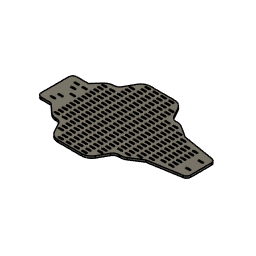
Old_Electronics plate v1 (Autodesk Fusion 360 design; units mm, degrees)
Autodesk Fusion 360 part; units mm, degrees
note: some values were not read from the file. Set by a fixed rule: which sketch regions a step uses.
(part 1 of 4)
sketch "Sketch2" plane through (0, 0, 0) normal (0, 1, 0) x (1, 0, 0)
  line L0 (270, -122.5) -> (360, -107.5)
  line L1 (360, -37.5) -> (270, -22.5)
  line L2 (360, -37.5) -> (360, -107.5)
  line L3 (270, -122.5) -> (235, -145)
  line L4 (235, 0) -> (270, -22.5)
  line L5 (-10, -27.5) -> (-10, -117.5)
  line L6 (55, -145) -> (25, -117.5)
  line L7 (25, -117.5) -> (-10, -117.5)
  line L8 (-10, -27.5) -> (29.7917, -27.5)
  line L9 (348.5, -55) -> (338.5, -55)
  line L10 (338.5, -58) -> (348.5, -58)
  arc A0 (338.5, -55) -> (338.5, -58) centre (338.5, -56.5) ccw
  arc A1 (348.5, -58) -> (348.5, -55) centre (348.5, -56.5) ccw
  line L11 (338.5, -87) -> (348.5, -87)
  arc A2 (338.5, -87) -> (338.5, -90) centre (338.5, -88.5) ccw
  line L12 (348.5, -90) -> (338.5, -90)
  arc A3 (348.5, -90) -> (348.5, -87) centre (348.5, -88.5) ccw
  line L13 (25, -55) -> (15, -55)
  arc A4 (15, -55) -> (15, -58) centre (15, -56.5) ccw
  line L14 (15, -58) -> (25, -58)
  arc A5 (25, -58) -> (25, -55) centre (25, -56.5) ccw
  line L15 (25, -90) -> (15, -90)
  line L16 (15, -87) -> (25, -87)
  arc A6 (25, -90) -> (25, -87) centre (25, -88.5) ccw
  arc A7 (15, -87) -> (15, -90) centre (15, -88.5) ccw
  line L17 (180, -71) -> (170, -71)
  line L18 (170, -74) -> (180, -74)
  arc A8 (170, -71) -> (170, -74) centre (170, -72.5) ccw
  arc A9 (180, -74) -> (180, -71) centre (180, -72.5) ccw
  arc A10 (120, -184) -> (120, -181) centre (120, -182.5) ccw
  line L19 (120, -181) -> (110, -181)
  line L20 (110, -184) -> (120, -184)
  arc A11 (110, -181) -> (110, -184) centre (110, -182.5) ccw
  arc A12 (140, -184) -> (140, -181) centre (140, -182.5) ccw
  line L21 (140, -181) -> (130, -181)
  line L22 (130, -184) -> (140, -184)
  arc A13 (130, -181) -> (130, -184) centre (130, -182.5) ccw
  arc A14 (160, -184) -> (160, -181) centre (160, -182.5) ccw
  line L23 (160, -181) -> (150, -181)
  line L24 (150, -184) -> (160, -184)
  arc A15 (150, -181) -> (150, -184) centre (150, -182.5) ccw
  arc A16 (180, -184) -> (180, -181) centre (180, -182.5) ccw
  line L25 (180, -181) -> (170, -181)
  line L26 (170, -184) -> (180, -184)
  arc A17 (170, -181) -> (170, -184) centre (170, -182.5) ccw
  arc A18 (120, -174) -> (120, -171) centre (120, -172.5) ccw
  line L27 (120, -171) -> (110, -171)
  line L28 (110, -174) -> (120, -174)
  arc A19 (110, -171) -> (110, -174) centre (110, -172.5) ccw
  arc A20 (140, -174) -> (140, -171) centre (140, -172.5) ccw
  line L29 (140, -171) -> (130, -171)
  line L30 (130, -174) -> (140, -174)
  arc A21 (130, -171) -> (130, -174) centre (130, -172.5) ccw
  arc A22 (160, -174) -> (160, -171) centre (160, -172.5) ccw
  line L31 (160, -171) -> (150, -171)
  line L32 (150, -174) -> (160, -174)
  arc A23 (150, -171) -> (150, -174) centre (150, -172.5) ccw
  arc A24 (180, -174) -> (180, -171) centre (180, -172.5) ccw
  line L33 (180, -171) -> (170, -171)
  line L34 (170, -174) -> (180, -174)
  arc A25 (170, -171) -> (170, -174) centre (170, -172.5) ccw
  arc A26 (100, -164) -> (100, -161) centre (100, -162.5) ccw
  line L35 (100, -161) -> (90, -161)
  line L36 (90, -164) -> (100, -164)
  arc A27 (90, -161) -> (90, -164) centre (90, -162.5) ccw
  arc A28 (120, -164) -> (120, -161) centre (120, -162.5) ccw
  line L37 (120, -161) -> (110, -161)
  line L38 (110, -164) -> (120, -164)
  arc A29 (110, -161) -> (110, -164) centre (110, -162.5) ccw
  arc A30 (140, -164) -> (140, -161) centre (140, -162.5) ccw
  line L39 (140, -161) -> (130, -161)
  line L40 (130, -164) -> (140, -164)
  arc A31 (130, -161) -> (130, -164) centre (130, -162.5) ccw
  arc A32 (160, -164) -> (160, -161) centre (160, -162.5) ccw
  line L41 (160, -161) -> (150, -161)
  line L42 (150, -164) -> (160, -164)
  arc A33 (150, -161) -> (150, -164) centre (150, -162.5) ccw
  arc A34 (180, -164) -> (180, -161) centre (180, -162.5) ccw
  line L43 (180, -161) -> (170, -161)
  line L44 (170, -164) -> (180, -164)
  arc A35 (170, -161) -> (170, -164) centre (170, -162.5) ccw
  arc A36 (200, -164) -> (200, -161) centre (200, -162.5) ccw
  line L45 (200, -161) -> (190, -161)
  line L46 (190, -164) -> (200, -164)
  arc A37 (190, -161) -> (190, -164) centre (190, -162.5) ccw
  arc A38 (100, -154) -> (100, -151) centre (100, -152.5) ccw
  line L47 (100, -151) -> (90, -151)
  line L48 (90, -154) -> (100, -154)
  arc A39 (90, -151) -> (90, -154) centre (90, -152.5) ccw
  arc A40 (120, -154) -> (120, -151) centre (120, -152.5) ccw
  line L49 (120, -151) -> (110, -151)
  line L50 (110, -154) -> (120, -154)
  arc A41 (110, -151) -> (110, -154) centre (110, -152.5) ccw
  arc A42 (140, -154) -> (140, -151) centre (140, -152.5) ccw
  line L51 (140, -151) -> (130, -151)
  line L52 (130, -154) -> (140, -154)
  arc A43 (130, -151) -> (130, -154) centre (130, -152.5) ccw
  arc A44 (160, -154) -> (160, -151) centre (160, -152.5) ccw
  line L53 (160, -151) -> (150, -151)
  line L54 (150, -154) -> (160, -154)
  arc A45 (150, -151) -> (150, -154) centre (150, -152.5) ccw
  arc A46 (180, -154) -> (180, -151) centre (180, -152.5) ccw
  line L55 (180, -151) -> (170, -151)
  line L56 (170, -154) -> (180, -154)
  arc A47 (170, -151) -> (170, -154) centre (170, -152.5) ccw
  arc A48 (200, -154) -> (200, -151) centre (200, -152.5) ccw
  line L57 (200, -151) -> (190, -151)
  line L58 (190, -154) -> (200, -154)
  arc A49 (190, -151) -> (190, -154) centre (190, -152.5) ccw
  arc A50 (100, -144) -> (100, -141) centre (100, -142.5) ccw
  line L59 (100, -141) -> (90, -141)
  line L60 (90, -144) -> (100, -144)
  arc A51 (90, -141) -> (90, -144) centre (90, -142.5) ccw
  arc A52 (120, -144) -> (120, -141) centre (120, -142.5) ccw
  line L61 (120, -141) -> (110, -141)
  line L62 (110, -144) -> (120, -144)
  arc A53 (110, -141) -> (110, -144) centre (110, -142.5) ccw
  arc A54 (140, -144) -> (140, -141) centre (140, -142.5) ccw
  line L63 (140, -141) -> (130, -141)
  line L64 (130, -144) -> (140, -144)
  arc A55 (130, -141) -> (130, -144) centre (130, -142.5) ccw
  arc A56 (160, -144) -> (160, -141) centre (160, -142.5) ccw
  line L65 (160, -141) -> (150, -141)
  line L66 (150, -144) -> (160, -144)
  arc A57 (150, -141) -> (150, -144) centre (150, -142.5) ccw
  arc A58 (180, -144) -> (180, -141) centre (180, -142.5) ccw
  line L67 (180, -141) -> (170, -141)
  line L68 (170, -144) -> (180, -144)
  arc A59 (170, -141) -> (170, -144) centre (170, -142.5) ccw
  arc A60 (200, -144) -> (200, -141) centre (200, -142.5) ccw
  line L69 (200, -141) -> (190, -141)
  line L70 (190, -144) -> (200, -144)
  arc A61 (190, -141) -> (190, -144) centre (190, -142.5) ccw
  arc A62 (60, -134) -> (60, -131) centre (60, -132.5) ccw
  line L71 (60, -131) -> (50, -131)
  line L72 (50, -134) -> (60, -134)
  arc A63 (50, -131) -> (50, -134) centre (50, -132.5) ccw
  arc A64 (80, -134) -> (80, -131) centre (80, -132.5) ccw
  line L73 (80, -131) -> (70, -131)
  line L74 (70, -134) -> (80, -134)
  arc A65 (70, -131) -> (70, -134) centre (70, -132.5) ccw
  arc A66 (100, -134) -> (100, -131) centre (100, -132.5) ccw
  line L75 (100, -131) -> (90, -131)
  line L76 (90, -134) -> (100, -134)
  arc A67 (90, -131) -> (90, -134) centre (90, -132.5) ccw
  arc A68 (120, -134) -> (120, -131) centre (120, -132.5) ccw
  line L77 (120, -131) -> (110, -131)
  line L78 (110, -134) -> (120, -134)
  arc A69 (110, -131) -> (110, -134) centre (110, -132.5) ccw
  arc A70 (140, -134) -> (140, -131) centre (140, -132.5) ccw
  line L79 (140, -131) -> (130, -131)
  line L80 (130, -134) -> (140, -134)
  arc A71 (130, -131) -> (130, -134) centre (130, -132.5) ccw
  arc A72 (160, -134) -> (160, -131) centre (160, -132.5) ccw
  line L81 (160, -131) -> (150, -131)
  line L82 (150, -134) -> (160, -134)
  arc A73 (150, -131) -> (150, -134) centre (150, -132.5) ccw
  arc A74 (180, -134) -> (180, -131) centre (180, -132.5) ccw
  line L83 (180, -131) -> (170, -131)
  line L84 (170, -134) -> (180, -134)
  arc A75 (170, -131) -> (170, -134) centre (170, -132.5) ccw
  arc A76 (200, -134) -> (200, -131) centre (200, -132.5) ccw
  line L85 (200, -131) -> (190, -131)
  line L86 (190, -134) -> (200, -134)
  arc A77 (190, -131) -> (190, -134) centre (190, -132.5) ccw
  arc A78 (220, -134) -> (220, -131) centre (220, -132.5) ccw
  line L87 (220, -131) -> (210, -131)
  line L88 (210, -134) -> (220, -134)
  arc A79 (210, -131) -> (210, -134) centre (210, -132.5) ccw
  arc A80 (240, -134) -> (240, -131) centre (240, -132.5) ccw
  line L89 (240, -131) -> (230, -131)
  line L90 (230, -134) -> (240, -134)
  arc A81 (230, -131) -> (230, -134) centre (230, -132.5) ccw
  arc A82 (60, -124) -> (60, -121) centre (60, -122.5) ccw
  line L91 (60, -121) -> (50, -121)
  line L92 (50, -124) -> (60, -124)
  arc A83 (50, -121) -> (50, -124) centre (50, -122.5) ccw
  arc A84 (80, -124) -> (80, -121) centre (80, -122.5) ccw
  line L93 (80, -121) -> (70, -121)
  line L94 (70, -124) -> (80, -124)
  arc A85 (70, -121) -> (70, -124) centre (70, -122.5) ccw
  arc A86 (100, -124) -> (100, -121) centre (100, -122.5) ccw
  line L95 (100, -121) -> (90, -121)
  line L96 (90, -124) -> (100, -124)
  arc A87 (90, -121) -> (90, -124) centre (90, -122.5) ccw
  arc A88 (120, -124) -> (120, -121) centre (120, -122.5) ccw
  line L97 (120, -121) -> (110, -121)
  line L98 (110, -124) -> (120, -124)
  arc A89 (110, -121) -> (110, -124) centre (110, -122.5) ccw
  arc A90 (140, -124) -> (140, -121) centre (140, -122.5) ccw
  line L99 (140, -121) -> (130, -121)
  line L100 (130, -124) -> (140, -124)
  arc A91 (130, -121) -> (130, -124) centre (130, -122.5) ccw
  arc A92 (160, -124) -> (160, -121) centre (160, -122.5) ccw
  line L101 (160, -121) -> (150, -121)
  line L102 (150, -124) -> (160, -124)
  arc A93 (150, -121) -> (150, -124) centre (150, -122.5) ccw
  arc A94 (180, -124) -> (180, -121) centre (180, -122.5) ccw
  line L103 (180, -121) -> (170, -121)
  line L104 (170, -124) -> (180, -124)
  arc A95 (170, -121) -> (170, -124) centre (170, -122.5) ccw
  arc A96 (200, -124) -> (200, -121) centre (200, -122.5) ccw
  line L105 (200, -121) -> (190, -121)
  line L106 (190, -124) -> (200, -124)
  arc A97 (190, -121) -> (190, -124) centre (190, -122.5) ccw
  arc A98 (220, -124) -> (220, -121) centre (220, -122.5) ccw
  line L107 (220, -121) -> (210, -121)
  line L108 (210, -124) -> (220, -124)
  arc A99 (210, -121) -> (210, -124) centre (210, -122.5) ccw
  arc A100 (240, -124) -> (240, -121) centre (240, -122.5) ccw
  line L109 (240, -121) -> (230, -121)
  line L110 (230, -124) -> (240, -124)
  arc A101 (230, -121) -> (230, -124) centre (230, -122.5) ccw
  arc A102 (260, -124) -> (260, -121) centre (260, -122.5) ccw
  line L111 (260, -121) -> (250, -121)
  line L112 (250, -124) -> (260, -124)
  arc A103 (250, -121) -> (250, -124) centre (250, -122.5) ccw
  arc A104 (60, -114) -> (60, -111) centre (60, -112.5) ccw
  line L113 (60, -111) -> (50, -111)
  line L114 (50, -114) -> (60, -114)
  arc A105 (50, -111) -> (50, -114) centre (50, -112.5) ccw
  arc A106 (80, -114) -> (80, -111) centre (80, -112.5) ccw
  line L115 (80, -111) -> (70, -111)
  line L116 (70, -114) -> (80, -114)
  arc A107 (70, -111) -> (70, -114) centre (70, -112.5) ccw
  arc A108 (100, -114) -> (100, -111) centre (100, -112.5) ccw
  line L117 (100, -111) -> (90, -111)
  line L118 (90, -114) -> (100, -114)
  arc A109 (90, -111) -> (90, -114) centre (90, -112.5) ccw
  arc A110 (120, -114) -> (120, -111) centre (120, -112.5) ccw
  line L119 (120, -111) -> (110, -111)
  line L120 (110, -114) -> (120, -114)
  arc A111 (110, -111) -> (110, -114) centre (110, -112.5) ccw
  arc A112 (140, -114) -> (140, -111) centre (140, -112.5) ccw
  line L121 (140, -111) -> (130, -111)
  line L122 (130, -114) -> (140, -114)
  arc A113 (130, -111) -> (130, -114) centre (130, -112.5) ccw
  arc A114 (160, -114) -> (160, -111) centre (160, -112.5) ccw
  line L123 (160, -111) -> (150, -111)
  line L124 (150, -114) -> (160, -114)
  arc A115 (150, -111) -> (150, -114) centre (150, -112.5) ccw
  arc A116 (180, -114) -> (180, -111) centre (180, -112.5) ccw
  line L125 (180, -111) -> (170, -111)
  line L126 (170, -114) -> (180, -114)
  arc A117 (170, -111) -> (170, -114) centre (170, -112.5) ccw
  arc A118 (200, -114) -> (200, -111) centre (200, -112.5) ccw
  line L127 (200, -111) -> (190, -111)
  line L128 (190, -114) -> (200, -114)
  arc A119 (190, -111) -> (190, -114) centre (190, -112.5) ccw
  arc A120 (220, -114) -> (220, -111) centre (220, -112.5) ccw
  line L129 (220, -111) -> (210, -111)
  line L130 (210, -114) -> (220, -114)
  arc A121 (210, -111) -> (210, -114) centre (210, -112.5) ccw
  arc A122 (240, -114) -> (240, -111) centre (240, -112.5) ccw
  line L131 (240, -111) -> (230, -111)
  line L132 (230, -114) -> (240, -114)
  arc A123 (230, -111) -> (230, -114) centre (230, -112.5) ccw
  arc A124 (260, -114) -> (260, -111) centre (260, -112.5) ccw
  line L133 (260, -111) -> (250, -111)
  line L134 (250, -114) -> (260, -114)
  arc A125 (250, -111) -> (250, -114) centre (250, -112.5) ccw
  arc A126 (280, -114) -> (280, -111) centre (280, -112.5) ccw
  line L135 (280, -111) -> (270, -111)
  line L136 (270, -114) -> (280, -114)
  arc A127 (270, -111) -> (270, -114) centre (270, -112.5) ccw
  arc A128 (20, -104) -> (20, -101) centre (20, -102.5) ccw
  line L137 (20, -101) -> (10, -101)
  line L138 (10, -104) -> (20, -104)
  arc A129 (10, -101) -> (10, -104) centre (10, -102.5) ccw
  arc A130 (60, -104) -> (60, -101) centre (60, -102.5) ccw
  line L139 (60, -101) -> (50, -101)
  line L140 (50, -104) -> (60, -104)
  arc A131 (50, -101) -> (50, -104) centre (50, -102.5) ccw
  arc A132 (80, -104) -> (80, -101) centre (80, -102.5) ccw
  line L141 (80, -101) -> (70, -101)
  line L142 (70, -104) -> (80, -104)
  arc A133 (70, -101) -> (70, -104) centre (70, -102.5) ccw
  arc A134 (100, -104) -> (100, -101) centre (100, -102.5) ccw
  line L143 (100, -101) -> (90, -101)
  line L144 (90, -104) -> (100, -104)
  arc A135 (90, -101) -> (90, -104) centre (90, -102.5) ccw
  arc A136 (120, -104) -> (120, -101) centre (120, -102.5) ccw
  line L145 (120, -101) -> (110, -101)
  line L146 (110, -104) -> (120, -104)
  arc A137 (110, -101) -> (110, -104) centre (110, -102.5) ccw
  arc A138 (140, -104) -> (140, -101) centre (140, -102.5) ccw
  line L147 (140, -101) -> (130, -101)
  line L148 (130, -104) -> (140, -104)
  arc A139 (130, -101) -> (130, -104) centre (130, -102.5) ccw
  arc A140 (160, -104) -> (160, -101) centre (160, -102.5) ccw
  line L149 (160, -101) -> (150, -101)
  line L150 (150, -104) -> (160, -104)
  arc A141 (150, -101) -> (150, -104) centre (150, -102.5) ccw
  arc A142 (180, -104) -> (180, -101) centre (180, -102.5) ccw
  line L151 (180, -101) -> (170, -101)
  line L152 (170, -104) -> (180, -104)
  arc A143 (170, -101) -> (170, -104) centre (170, -102.5) ccw
  arc A144 (200, -104) -> (200, -101) centre (200, -102.5) ccw
  line L153 (200, -101) -> (190, -101)
  line L154 (190, -104) -> (200, -104)
  arc A145 (190, -101) -> (190, -104) centre (190, -102.5) ccw
  arc A146 (220, -104) -> (220, -101) centre (220, -102.5) ccw
  line L155 (220, -101) -> (210, -101)
  line L156 (210, -104) -> (220, -104)
  arc A147 (210, -101) -> (210, -104) centre (210, -102.5) ccw
  arc A148 (240, -104) -> (240, -101) centre (240, -102.5) ccw
  line L157 (240, -101) -> (230, -101)
  line L158 (230, -104) -> (240, -104)
  arc A149 (230, -101) -> (230, -104) centre (230, -102.5) ccw
  arc A150 (260, -104) -> (260, -101) centre (260, -102.5) ccw
  line L159 (260, -101) -> (250, -101)
  line L160 (250, -104) -> (260, -104)
  arc A151 (250, -101) -> (250, -104) centre (250, -102.5) ccw
  arc A152 (280, -104) -> (280, -101) centre (280, -102.5) ccw
  line L161 (280, -101) -> (270, -101)
  line L162 (270, -104) -> (280, -104)
  arc A153 (270, -101) -> (270, -104) centre (270, -102.5) ccw
  arc A154 (300, -104) -> (300, -101) centre (300, -102.5) ccw
  line L163 (300, -101) -> (290, -101)
  line L164 (290, -104) -> (300, -104)
  arc A155 (290, -101) -> (290, -104) centre (290, -102.5) ccw
  arc A156 (320, -104) -> (320, -101) centre (320, -102.5) ccw
  line L165 (320, -101) -> (310, -101)
  line L166 (310, -104) -> (320, -104)
  arc A157 (310, -101) -> (310, -104) centre (310, -102.5) ccw
  arc A158 (60, -94) -> (60, -91) centre (60, -92.5) ccw
  line L167 (60, -91) -> (50, -91)
  line L168 (50, -94) -> (60, -94)
  arc A159 (50, -91) -> (50, -94) centre (50, -92.5) ccw
  arc A160 (80, -94) -> (80, -91) centre (80, -92.5) ccw
  line L169 (80, -91) -> (70, -91)
  line L170 (70, -94) -> (80, -94)
  arc A161 (70, -91) -> (70, -94) centre (70, -92.5) ccw
  arc A162 (100, -94) -> (100, -91) centre (100, -92.5) ccw
  line L171 (100, -91) -> (90, -91)
  line L172 (90, -94) -> (100, -94)
  arc A163 (90, -91) -> (90, -94) centre (90, -92.5) ccw
  arc A164 (120, -94) -> (120, -91) centre (120, -92.5) ccw
  line L173 (120, -91) -> (110, -91)
  line L174 (110, -94) -> (120, -94)
  arc A165 (110, -91) -> (110, -94) centre (110, -92.5) ccw
  arc A166 (140, -94) -> (140, -91) centre (140, -92.5) ccw
  line L175 (140, -91) -> (130, -91)
  line L176 (130, -94) -> (140, -94)
  arc A167 (130, -91) -> (130, -94) centre (130, -92.5) ccw
  arc A168 (160, -94) -> (160, -91) centre (160, -92.5) ccw
  line L177 (160, -91) -> (150, -91)
  line L178 (150, -94) -> (160, -94)
  arc A169 (150, -91) -> (150, -94) centre (150, -92.5) ccw
  arc A170 (180, -94) -> (180, -91) centre (180, -92.5) ccw
  line L179 (180, -91) -> (170, -91)
  line L180 (170, -94) -> (180, -94)
  arc A171 (170, -91) -> (170, -94) centre (170, -92.5) ccw
  arc A172 (200, -94) -> (200, -91) centre (200, -92.5) ccw
  line L181 (200, -91) -> (190, -91)
  line L182 (190, -94) -> (200, -94)
  arc A173 (190, -91) -> (190, -94) centre (190, -92.5) ccw
  arc A174 (220, -94) -> (220, -91) centre (220, -92.5) ccw
  line L183 (220, -91) -> (210, -91)
  line L184 (210, -94) -> (220, -94)
  arc A175 (210, -91) -> (210, -94) centre (210, -92.5) ccw
  arc A176 (240, -94) -> (240, -91) centre (240, -92.5) ccw
  line L185 (240, -91) -> (230, -91)
  line L186 (230, -94) -> (240, -94)
  arc A177 (230, -91) -> (230, -94) centre (230, -92.5) ccw
  arc A178 (260, -94) -> (260, -91) centre (260, -92.5) ccw
  line L187 (260, -91) -> (250, -91)
  line L188 (250, -94) -> (260, -94)
  arc A179 (250, -91) -> (250, -94) centre (250, -92.5) ccw
  arc A180 (280, -94) -> (280, -91) centre (280, -92.5) ccw
  line L189 (280, -91) -> (270, -91)
  line L190 (270, -94) -> (280, -94)
  arc A181 (270, -91) -> (270, -94) centre (270, -92.5) ccw
  arc A182 (300, -94) -> (300, -91) centre (300, -92.5) ccw
  line L191 (300, -91) -> (290, -91)
  line L192 (290, -94) -> (300, -94)
  arc A183 (290, -91) -> (290, -94) centre (290, -92.5) ccw
  arc A184 (320, -94) -> (320, -91) centre (320, -92.5) ccw
  line L193 (320, -91) -> (310, -91)
  line L194 (310, -94) -> (320, -94)
  arc A185 (310, -91) -> (310, -94) centre (310, -92.5) ccw
  arc A186 (60, -84) -> (60, -81) centre (60, -82.5) ccw
  line L195 (60, -81) -> (50, -81)
  line L196 (50, -84) -> (60, -84)
  arc A187 (50, -81) -> (50, -84) centre (50, -82.5) ccw
  arc A188 (80, -84) -> (80, -81) centre (80, -82.5) ccw
  line L197 (80, -81) -> (70, -81)
  line L198 (70, -84) -> (80, -84)
  arc A189 (70, -81) -> (70, -84) centre (70, -82.5) ccw
  arc A190 (100, -84) -> (100, -81) centre (100, -82.5) ccw
  line L199 (100, -81) -> (90, -81)
  line L200 (90, -84) -> (100, -84)
  arc A191 (90, -81) -> (90, -84) centre (90, -82.5) ccw
  arc A192 (120, -84) -> (120, -81) centre (120, -82.5) ccw
  line L201 (120, -81) -> (110, -81)
  line L202 (110, -84) -> (120, -84)
  arc A193 (110, -81) -> (110, -84) centre (110, -82.5) ccw
  arc A194 (140, -84) -> (140, -81) centre (140, -82.5) ccw
  line L203 (140, -81) -> (130, -81)
  line L204 (130, -84) -> (140, -84)
  arc A195 (130, -81) -> (130, -84) centre (130, -82.5) ccw
  arc A196 (160, -84) -> (160, -81) centre (160, -82.5) ccw
  line L205 (160, -81) -> (150, -81)
  line L206 (150, -84) -> (160, -84)
  arc A197 (150, -81) -> (150, -84) centre (150, -82.5) ccw
  arc A198 (180, -84) -> (180, -81) centre (180, -82.5) ccw
  line L207 (180, -81) -> (170, -81)
  line L208 (170, -84) -> (180, -84)
  arc A199 (170, -81) -> (170, -84) centre (170, -82.5) ccw
  arc A200 (200, -84) -> (200, -81) centre (200, -82.5) ccw
  line L209 (200, -81) -> (190, -81)
  line L210 (190, -84) -> (200, -84)
  arc A201 (190, -81) -> (190, -84) centre (190, -82.5) ccw
  arc A202 (220, -84) -> (220, -81) centre (220, -82.5) ccw
  line L211 (220, -81) -> (210, -81)
  line L212 (210, -84) -> (220, -84)
  arc A203 (210, -81) -> (210, -84) centre (210, -82.5) ccw
  arc A204 (240, -84) -> (240, -81) centre (240, -82.5) ccw
  line L213 (240, -81) -> (230, -81)
  line L214 (230, -84) -> (240, -84)
  arc A205 (230, -81) -> (230, -84) centre (230, -82.5) ccw
  arc A206 (260, -84) -> (260, -81) centre (260, -82.5) ccw
  line L215 (260, -81) -> (250, -81)
  line L216 (250, -84) -> (260, -84)
  arc A207 (250, -81) -> (250, -84) centre (250, -82.5) ccw
  arc A208 (280, -84) -> (280, -81) centre (280, -82.5) ccw
  line L217 (280, -81) -> (270, -81)
  line L218 (270, -84) -> (280, -84)
  arc A209 (270, -81) -> (270, -84) centre (270, -82.5) ccw
  arc A210 (300, -84) -> (300, -81) centre (300, -82.5) ccw
  line L219 (300, -81) -> (290, -81)
  line L220 (290, -84) -> (300, -84)
  arc A211 (290, -81) -> (290, -84) centre (290, -82.5) ccw
  arc A212 (320, -84) -> (320, -81) centre (320, -82.5) ccw
  line L221 (320, -81) -> (310, -81)
  line L222 (310, -84) -> (320, -84)
  arc A213 (310, -81) -> (310, -84) centre (310, -82.5) ccw
  arc A214 (40, -74) -> (40, -71) centre (40, -72.5) ccw
  line L223 (40, -71) -> (30, -71)
  line L224 (30, -74) -> (40, -74)
  arc A215 (30, -71) -> (30, -74) centre (30, -72.5) ccw
  arc A216 (60, -74) -> (60, -71) centre (60, -72.5) ccw
  line L225 (60, -71) -> (50, -71)
  line L226 (50, -74) -> (60, -74)
  arc A217 (50, -71) -> (50, -74) centre (50, -72.5) ccw
  arc A218 (80, -74) -> (80, -71) centre (80, -72.5) ccw
  line L227 (80, -71) -> (70, -71)
  line L228 (70, -74) -> (80, -74)
  arc A219 (70, -71) -> (70, -74) centre (70, -72.5) ccw
  arc A220 (100, -74) -> (100, -71) centre (100, -72.5) ccw
  line L229 (100, -71) -> (90, -71)
  line L230 (90, -74) -> (100, -74)
  arc A221 (90, -71) -> (90, -74) centre (90, -72.5) ccw
  arc A222 (120, -74) -> (120, -71) centre (120, -72.5) ccw
  line L231 (120, -71) -> (110, -71)
  line L232 (110, -74) -> (120, -74)
  arc A223 (110, -71) -> (110, -74) centre (110, -72.5) ccw
  arc A224 (140, -74) -> (140, -71) centre (140, -72.5) ccw
  line L233 (140, -71) -> (130, -71)
  line L234 (130, -74) -> (140, -74)
  arc A225 (130, -71) -> (130, -74) centre (130, -72.5) ccw
  arc A226 (160, -74) -> (160, -71) centre (160, -72.5) ccw
  line L235 (160, -71) -> (150, -71)
  line L236 (150, -74) -> (160, -74)
  arc A227 (150, -71) -> (150, -74) centre (150, -72.5) ccw
  arc A228 (200, -74) -> (200, -71) centre (200, -72.5) ccw
  line L237 (200, -71) -> (190, -71)
  line L238 (190, -74) -> (200, -74)
  arc A229 (190, -71) -> (190, -74) centre (190, -72.5) ccw
  arc A230 (220, -74) -> (220, -71) centre (220, -72.5) ccw
  line L239 (220, -71) -> (210, -71)
  line L240 (210, -74) -> (220, -74)
  arc A231 (210, -71) -> (210, -74) centre (210, -72.5) ccw
  arc A232 (240, -74) -> (240, -71) centre (240, -72.5) ccw
  line L241 (240, -71) -> (230, -71)
  line L242 (230, -74) -> (240, -74)
  arc A233 (230, -71) -> (230, -74) centre (230, -72.5) ccw
  arc A234 (260, -74) -> (260, -71) centre (260, -72.5) ccw
  line L243 (260, -71) -> (250, -71)
  line L244 (250, -74) -> (260, -74)
  arc A235 (250, -71) -> (250, -74) centre (250, -72.5) ccw
  arc A236 (280, -74) -> (280, -71) centre (280, -72.5) ccw
  line L245 (280, -71) -> (270, -71)
  line L246 (270, -74) -> (280, -74)
  arc A237 (270, -71) -> (270, -74) centre (270, -72.5) ccw
  arc A238 (300, -74) -> (300, -71) centre (300, -72.5) ccw
  line L247 (300, -71) -> (290, -71)
  line L248 (290, -74) -> (300, -74)
  arc A239 (290, -71) -> (290, -74) centre (290, -72.5) ccw
  arc A240 (320, -74) -> (320, -71) centre (320, -72.5) ccw
  line L249 (320, -71) -> (310, -71)
  line L250 (310, -74) -> (320, -74)
  arc A241 (310, -71) -> (310, -74) centre (310, -72.5) ccw
  arc A242 (60, -64) -> (60, -61) centre (60, -62.5) ccw
  line L251 (60, -61) -> (50, -61)
  line L252 (50, -64) -> (60, -64)
  arc A243 (50, -61) -> (50, -64) centre (50, -62.5) ccw
  arc A244 (80, -64) -> (80, -61) centre (80, -62.5) ccw
  line L253 (80, -61) -> (70, -61)
  line L254 (70, -64) -> (80, -64)
  arc A245 (70, -61) -> (70, -64) centre (70, -62.5) ccw
  arc A246 (100, -64) -> (100, -61) centre (100, -62.5) ccw
  line L255 (100, -61) -> (90, -61)
  line L256 (90, -64) -> (100, -64)
  arc A247 (90, -61) -> (90, -64) centre (90, -62.5) ccw
  arc A248 (120, -64) -> (120, -61) centre (120, -62.5) ccw
  line L257 (120, -61) -> (110, -61)
  line L258 (110, -64) -> (120, -64)
  arc A249 (110, -61) -> (110, -64) centre (110, -62.5) ccw
  arc A250 (140, -64) -> (140, -61) centre (140, -62.5) ccw
  line L259 (140, -61) -> (130, -61)
  line L260 (130, -64) -> (140, -64)
  arc A251 (130, -61) -> (130, -64) centre (130, -62.5) ccw
  arc A252 (160, -64) -> (160, -61) centre (160, -62.5) ccw
  line L261 (160, -61) -> (150, -61)
  line L262 (150, -64) -> (160, -64)
  arc A253 (150, -61) -> (150, -64) centre (150, -62.5) ccw
  arc A254 (180, -64) -> (180, -61) centre (180, -62.5) ccw
  line L263 (180, -61) -> (170, -61)
  line L264 (170, -64) -> (180, -64)
  arc A255 (170, -61) -> (170, -64) centre (170, -62.5) ccw
  arc A256 (200, -64) -> (200, -61) centre (200, -62.5) ccw
  line L265 (200, -61) -> (190, -61)
  line L266 (190, -64) -> (200, -64)
  arc A257 (190, -61) -> (190, -64) centre (190, -62.5) ccw
  arc A258 (220, -64) -> (220, -61) centre (220, -62.5) ccw
  line L267 (220, -61) -> (210, -61)
  line L268 (210, -64) -> (220, -64)
  arc A259 (210, -61) -> (210, -64) centre (210, -62.5) ccw
  arc A260 (240, -64) -> (240, -61) centre (240, -62.5) ccw
  line L269 (240, -61) -> (230, -61)
  line L270 (230, -64) -> (240, -64)
  arc A261 (230, -61) -> (230, -64) centre (230, -62.5) ccw
  arc A262 (260, -64) -> (260, -61) centre (260, -62.5) ccw
  line L271 (260, -61) -> (250, -61)
  line L272 (250, -64) -> (260, -64)
  arc A263 (250, -61) -> (250, -64) centre (250, -62.5) ccw
  arc A264 (280, -64) -> (280, -61) centre (280, -62.5) ccw
  line L273 (280, -61) -> (270, -61)
  line L274 (270, -64) -> (280, -64)
  arc A265 (270, -61) -> (270, -64) centre (270, -62.5) ccw
  arc A266 (300, -64) -> (300, -61) centre (300, -62.5) ccw
  line L275 (300, -61) -> (290, -61)
  line L276 (290, -64) -> (300, -64)
  arc A267 (290, -61) -> (290, -64) centre (290, -62.5) ccw
  arc A268 (320, -64) -> (320, -61) centre (320, -62.5) ccw
  line L277 (320, -61) -> (310, -61)
  line L278 (310, -64) -> (320, -64)
  arc A269 (310, -61) -> (310, -64) centre (310, -62.5) ccw
  arc A270 (60, -54) -> (60, -51) centre (60, -52.5) ccw
  line L279 (60, -51) -> (50, -51)
  line L280 (50, -54) -> (60, -54)
  arc A271 (50, -51) -> (50, -54) centre (50, -52.5) ccw
  arc A272 (80, -54) -> (80, -51) centre (80, -52.5) ccw
  line L281 (80, -51) -> (70, -51)
  line L282 (70, -54) -> (80, -54)
  arc A273 (70, -51) -> (70, -54) centre (70, -52.5) ccw
  arc A274 (100, -54) -> (100, -51) centre (100, -52.5) ccw
  line L283 (100, -51) -> (90, -51)
  line L284 (90, -54) -> (100, -54)
  arc A275 (90, -51) -> (90, -54) centre (90, -52.5) ccw
  arc A276 (120, -54) -> (120, -51) centre (120, -52.5) ccw
  line L285 (120, -51) -> (110, -51)
  line L286 (110, -54) -> (120, -54)
  arc A277 (110, -51) -> (110, -54) centre (110, -52.5) ccw
  arc A278 (140, -54) -> (140, -51) centre (140, -52.5) ccw
  line L287 (140, -51) -> (130, -51)
  line L288 (130, -54) -> (140, -54)
  arc A279 (130, -51) -> (130, -54) centre (130, -52.5) ccw
  arc A280 (160, -54) -> (160, -51) centre (160, -52.5) ccw
  line L289 (160, -51) -> (150, -51)
  line L290 (150, -54) -> (160, -54)
  arc A281 (150, -51) -> (150, -54) centre (150, -52.5) ccw
  arc A282 (180, -54) -> (180, -51) centre (180, -52.5) ccw
  line L291 (180, -51) -> (170, -51)
  line L292 (170, -54) -> (180, -54)
  arc A283 (170, -51) -> (170, -54) centre (170, -52.5) ccw
  arc A284 (200, -54) -> (200, -51) centre (200, -52.5) ccw
  line L293 (200, -51) -> (190, -51)
  line L294 (190, -54) -> (200, -54)
  arc A285 (190, -51) -> (190, -54) centre (190, -52.5) ccw
  arc A286 (220, -54) -> (220, -51) centre (220, -52.5) ccw
  line L295 (220, -51) -> (210, -51)
  line L296 (210, -54) -> (220, -54)
  arc A287 (210, -51) -> (210, -54) centre (210, -52.5) ccw
  arc A288 (240, -54) -> (240, -51) centre (240, -52.5) ccw
  line L297 (240, -51) -> (230, -51)
  line L298 (230, -54) -> (240, -54)
  arc A289 (230, -51) -> (230, -54) centre (230, -52.5) ccw
  arc A290 (260, -54) -> (260, -51) centre (260, -52.5) ccw
  line L299 (260, -51) -> (250, -51)
  line L300 (250, -54) -> (260, -54)
  arc A291 (250, -51) -> (250, -54) centre (250, -52.5) ccw
  arc A292 (280, -54) -> (280, -51) centre (280, -52.5) ccw
  line L301 (280, -51) -> (270, -51)
  line L302 (270, -54) -> (280, -54)
  arc A293 (270, -51) -> (270, -54) centre (270, -52.5) ccw
  arc A294 (300, -54) -> (300, -51) centre (300, -52.5) ccw
  line L303 (300, -51) -> (290, -51)
  line L304 (290, -54) -> (300, -54)
  arc A295 (290, -51) -> (290, -54) centre (290, -52.5) ccw
  arc A296 (320, -54) -> (320, -51) centre (320, -52.5) ccw
  line L305 (320, -51) -> (310, -51)
  line L306 (310, -54) -> (320, -54)
  arc A297 (310, -51) -> (310, -54) centre (310, -52.5) ccw
  arc A298 (20, -44) -> (20, -41) centre (20, -42.5) ccw
  line L307 (20, -41) -> (10, -41)
  line L308 (10, -44) -> (20, -44)
  arc A299 (10, -41) -> (10, -44) centre (10, -42.5) ccw
  arc A300 (40, -44) -> (40, -41) centre (40, -42.5) ccw
  line L309 (40, -41) -> (30, -41)
  line L310 (30, -44) -> (40, -44)
  arc A301 (30, -41) -> (30, -44) centre (30, -42.5) ccw
  arc A302 (60, -44) -> (60, -41) centre (60, -42.5) ccw
  line L311 (60, -41) -> (50, -41)
  line L312 (50, -44) -> (60, -44)
  arc A303 (50, -41) -> (50, -44) centre (50, -42.5) ccw
  arc A304 (80, -44) -> (80, -41) centre (80, -42.5) ccw
  line L313 (80, -41) -> (70, -41)
  line L314 (70, -44) -> (80, -44)
  arc A305 (70, -41) -> (70, -44) centre (70, -42.5) ccw
  arc A306 (100, -44) -> (100, -41) centre (100, -42.5) ccw
  line L315 (100, -41) -> (90, -41)
  line L316 (90, -44) -> (100, -44)
  arc A307 (90, -41) -> (90, -44) centre (90, -42.5) ccw
  arc A308 (120, -44) -> (120, -41) centre (120, -42.5) ccw
  line L317 (120, -41) -> (110, -41)
  line L318 (110, -44) -> (120, -44)
  arc A309 (110, -41) -> (110, -44) centre (110, -42.5) ccw
  arc A310 (140, -44) -> (140, -41) centre (140, -42.5) ccw
  line L319 (140, -41) -> (130, -41)
  line L320 (130, -44) -> (140, -44)
  arc A311 (130, -41) -> (130, -44) centre (130, -42.5) ccw
  arc A312 (160, -44) -> (160, -41) centre (160, -42.5) ccw
  line L321 (160, -41) -> (150, -41)
  line L322 (150, -44) -> (160, -44)
  arc A313 (150, -41) -> (150, -44) centre (150, -42.5) ccw
  arc A314 (180, -44) -> (180, -41) centre (180, -42.5) ccw
  line L323 (180, -41) -> (170, -41)
  line L324 (170, -44) -> (180, -44)
  arc A315 (170, -41) -> (170, -44) centre (170, -42.5) ccw
  arc A316 (200, -44) -> (200, -41) centre (200, -42.5) ccw
  line L325 (200, -41) -> (190, -41)
  line L326 (190, -44) -> (200, -44)
  arc A317 (190, -41) -> (190, -44) centre (190, -42.5) ccw
  arc A318 (220, -44) -> (220, -41) centre (220, -42.5) ccw
  line L327 (220, -41) -> (210, -41)
  line L328 (210, -44) -> (220, -44)
  arc A319 (210, -41) -> (210, -44) centre (210, -42.5) ccw
  arc A320 (240, -44) -> (240, -41) centre (240, -42.5) ccw
  line L329 (240, -41) -> (230, -41)
  line L330 (230, -44) -> (240, -44)
  arc A321 (230, -41) -> (230, -44) centre (230, -42.5) ccw
  arc A322 (260, -44) -> (260, -41) centre (260, -42.5) ccw
  line L331 (260, -41) -> (250, -41)
  line L332 (250, -44) -> (260, -44)
  arc A323 (250, -41) -> (250, -44) centre (250, -42.5) ccw
  arc A324 (280, -44) -> (280, -41) centre (280, -42.5) ccw
  line L333 (280, -41) -> (270, -41)
  line L334 (270, -44) -> (280, -44)
  arc A325 (270, -41) -> (270, -44) centre (270, -42.5) ccw
  arc A326 (300, -44) -> (300, -41) centre (300, -42.5) ccw
  line L335 (300, -41) -> (290, -41)
  line L336 (290, -44) -> (300, -44)
  arc A327 (290, -41) -> (290, -44) centre (290, -42.5) ccw
  arc A328 (320, -44) -> (320, -41) centre (320, -42.5) ccw
  line L337 (320, -41) -> (310, -41)
  line L338 (310, -44) -> (320, -44)
  arc A329 (310, -41) -> (310, -44) centre (310, -42.5) ccw
  arc A330 (60, -34) -> (60, -31) centre (60, -32.5) ccw
  line L339 (60, -31) -> (50, -31)
  line L340 (50, -34) -> (60, -34)
  arc A331 (50, -31) -> (50, -34) centre (50, -32.5) ccw
  arc A332 (80, -34) -> (80, -31) centre (80, -32.5) ccw
  line L341 (80, -31) -> (70, -31)
  line L342 (70, -34) -> (80, -34)
  arc A333 (70, -31) -> (70, -34) centre (70, -32.5) ccw
  arc A334 (100, -34) -> (100, -31) centre (100, -32.5) ccw
  line L343 (100, -31) -> (90, -31)
  line L344 (90, -34) -> (100, -34)
  arc A335 (90, -31) -> (90, -34) centre (90, -32.5) ccw
  arc A336 (120, -34) -> (120, -31) centre (120, -32.5) ccw
  line L345 (120, -31) -> (110, -31)
  line L346 (110, -34) -> (120, -34)
  arc A337 (110, -31) -> (110, -34) centre (110, -32.5) ccw
  arc A338 (140, -34) -> (140, -31) centre (140, -32.5) ccw
  line L347 (140, -31) -> (130, -31)
  line L348 (130, -34) -> (140, -34)
  arc A339 (130, -31) -> (130, -34) centre (130, -32.5) ccw
  arc A340 (160, -34) -> (160, -31) centre (160, -32.5) ccw
  line L349 (160, -31) -> (150, -31)
  line L350 (150, -34) -> (160, -34)
  arc A341 (150, -31) -> (150, -34) centre (150, -32.5) ccw
  arc A342 (180, -34) -> (180, -31) centre (180, -32.5) ccw
  line L351 (180, -31) -> (170, -31)
  line L352 (170, -34) -> (180, -34)
  arc A343 (170, -31) -> (170, -34) centre (170, -32.5) ccw
  arc A344 (200, -34) -> (200, -31) centre (200, -32.5) ccw
  line L353 (200, -31) -> (190, -31)
  line L354 (190, -34) -> (200, -34)
  arc A345 (190, -31) -> (190, -34) centre (190, -32.5) ccw
  arc A346 (220, -34) -> (220, -31) centre (220, -32.5) ccw
  line L355 (220, -31) -> (210, -31)
  line L356 (210, -34) -> (220, -34)
  arc A347 (210, -31) -> (210, -34) centre (210, -32.5) ccw
  arc A348 (240, -34) -> (240, -31) centre (240, -32.5) ccw
  line L357 (240, -31) -> (230, -31)
  line L358 (230, -34) -> (240, -34)
  arc A349 (230, -31) -> (230, -34) centre (230, -32.5) ccw
  arc A350 (260, -34) -> (260, -31) centre (260, -32.5) ccw
  line L359 (260, -31) -> (250, -31)
  line L360 (250, -34) -> (260, -34)
  arc A351 (250, -31) -> (250, -34) centre (250, -32.5) ccw
  arc A352 (280, -34) -> (280, -31) centre (280, -32.5) ccw
  line L361 (280, -31) -> (270, -31)
  line L362 (270, -34) -> (280, -34)
  arc A353 (270, -31) -> (270, -34) centre (270, -32.5) ccw
  arc A354 (60, -24) -> (60, -21) centre (60, -22.5) ccw
  line L363 (60, -21) -> (50, -21)
  line L364 (50, -24) -> (60, -24)
  arc A355 (50, -21) -> (50, -24) centre (50, -22.5) ccw
  arc A356 (80, -24) -> (80, -21) centre (80, -22.5) ccw
  line L365 (80, -21) -> (70, -21)
  line L366 (70, -24) -> (80, -24)
  arc A357 (70, -21) -> (70, -24) centre (70, -22.5) ccw
  arc A358 (100, -24) -> (100, -21) centre (100, -22.5) ccw
  line L367 (100, -21) -> (90, -21)
  line L368 (90, -24) -> (100, -24)
  arc A359 (90, -21) -> (90, -24) centre (90, -22.5) ccw
  arc A360 (120, -24) -> (120, -21) centre (120, -22.5) ccw
  line L369 (120, -21) -> (110, -21)
  line L370 (110, -24) -> (120, -24)
  arc A361 (110, -21) -> (110, -24) centre (110, -22.5) ccw
  arc A362 (140, -24) -> (140, -21) centre (140, -22.5) ccw
  line L371 (140, -21) -> (130, -21)
  line L372 (130, -24) -> (140, -24)
  arc A363 (130, -21) -> (130, -24) centre (130, -22.5) ccw
  arc A364 (160, -24) -> (160, -21) centre (160, -22.5) ccw
  line L373 (160, -21) -> (150, -21)
  line L374 (150, -24) -> (160, -24)
  arc A365 (150, -21) -> (150, -24) centre (150, -22.5) ccw
  arc A366 (180, -24) -> (180, -21) centre (180, -22.5) ccw
  line L375 (180, -21) -> (170, -21)
  line L376 (170, -24) -> (180, -24)
  arc A367 (170, -21) -> (170, -24) centre (170, -22.5) ccw
  arc A368 (200, -24) -> (200, -21) centre (200, -22.5) ccw
  line L377 (200, -21) -> (190, -21)
  line L378 (190, -24) -> (200, -24)
  arc A369 (190, -21) -> (190, -24) centre (190, -22.5) ccw
  arc A370 (220, -24) -> (220, -21) centre (220, -22.5) ccw
  line L379 (220, -21) -> (210, -21)
  line L380 (210, -24) -> (220, -24)
  arc A371 (210, -21) -> (210, -24) centre (210, -22.5) ccw
  arc A372 (240, -24) -> (240, -21) centre (240, -22.5) ccw
  line L381 (240, -21) -> (230, -21)
  line L382 (230, -24) -> (240, -24)
  arc A373 (230, -21) -> (230, -24) centre (230, -22.5) ccw
  arc A374 (260, -24) -> (260, -21) centre (260, -22.5) ccw
  line L383 (260, -21) -> (250, -21)
  line L384 (250, -24) -> (260, -24)
  arc A375 (250, -21) -> (250, -24) centre (250, -22.5) ccw
  arc A376 (60, -14) -> (60, -11) centre (60, -12.5) ccw
  line L385 (60, -11) -> (50, -11)
  line L386 (50, -14) -> (60, -14)
  arc A377 (50, -11) -> (50, -14) centre (50, -12.5) ccw
  arc A378 (80, -14) -> (80, -11) centre (80, -12.5) ccw
  line L387 (80, -11) -> (70, -11)
  line L388 (70, -14) -> (80, -14)
  arc A379 (70, -11) -> (70, -14) centre (70, -12.5) ccw
  arc A380 (100, -14) -> (100, -11) centre (100, -12.5) ccw
  line L389 (100, -11) -> (90, -11)
  line L390 (90, -14) -> (100, -14)
  arc A381 (90, -11) -> (90, -14) centre (90, -12.5) ccw
  arc A382 (120, -14) -> (120, -11) centre (120, -12.5) ccw
  line L391 (120, -11) -> (110, -11)
  line L392 (110, -14) -> (120, -14)
  arc A383 (110, -11) -> (110, -14) centre (110, -12.5) ccw
  arc A384 (140, -14) -> (140, -11) centre (140, -12.5) ccw
  line L393 (140, -11) -> (130, -11)
  line L394 (130, -14) -> (140, -14)
  arc A385 (130, -11) -> (130, -14) centre (130, -12.5) ccw
  arc A386 (160, -14) -> (160, -11) centre (160, -12.5) ccw
  line L395 (160, -11) -> (150, -11)
  line L396 (150, -14) -> (160, -14)
  arc A387 (150, -11) -> (150, -14) centre (150, -12.5) ccw
  arc A388 (180, -14) -> (180, -11) centre (180, -12.5) ccw
  line L397 (180, -11) -> (170, -11)
  line L398 (170, -14) -> (180, -14)
  arc A389 (170, -11) -> (170, -14) centre (170, -12.5) ccw
  arc A390 (200, -14) -> (200, -11) centre (200, -12.5) ccw
  line L399 (200, -11) -> (190, -11)
  line L400 (190, -14) -> (200, -14)
  arc A391 (190, -11) -> (190, -14) centre (190, -12.5) ccw
  arc A392 (220, -14) -> (220, -11) centre (220, -12.5) ccw
  line L401 (220, -11) -> (210, -11)
  line L402 (210, -14) -> (220, -14)
  arc A393 (210, -11) -> (210, -14) centre (210, -12.5) ccw
  arc A394 (240, -14) -> (240, -11) centre (240, -12.5) ccw
  line L403 (240, -11) -> (230, -11)
  line L404 (230, -14) -> (240, -14)
  arc A395 (230, -11) -> (230, -14) centre (230, -12.5) ccw
  arc A396 (100, -4) -> (100, -1) centre (100, -2.5) ccw
  line L405 (100, -1) -> (90, -1)
  line L406 (90, -4) -> (100, -4)
  arc A397 (90, -1) -> (90, -4) centre (90, -2.5) ccw
  arc A398 (120, -4) -> (120, -1) centre (120, -2.5) ccw
  line L407 (120, -1) -> (110, -1)
  line L408 (110, -4) -> (120, -4)
  arc A399 (110, -1) -> (110, -4) centre (110, -2.5) ccw
  arc A400 (140, -4) -> (140, -1) centre (140, -2.5) ccw
  line L409 (140, -1) -> (130, -1)
  line L410 (130, -4) -> (140, -4)
  arc A401 (130, -1) -> (130, -4) centre (130, -2.5) ccw
  arc A402 (160, -4) -> (160, -1) centre (160, -2.5) ccw
  line L411 (160, -1) -> (150, -1)
  line L412 (150, -4) -> (160, -4)
  arc A403 (150, -1) -> (150, -4) centre (150, -2.5) ccw
  arc A404 (180, -4) -> (180, -1) centre (180, -2.5) ccw
  line L413 (180, -1) -> (170, -1)
  line L414 (170, -4) -> (180, -4)
  arc A405 (170, -1) -> (170, -4) centre (170, -2.5) ccw
  arc A406 (200, -4) -> (200, -1) centre (200, -2.5) ccw
  line L415 (200, -1) -> (190, -1)
  line L416 (190, -4) -> (200, -4)
  arc A407 (190, -1) -> (190, -4) centre (190, -2.5) ccw
  arc A408 (100, 6) -> (100, 9) centre (100, 7.5) ccw
  line L417 (100, 9) -> (90, 9)
  line L418 (90, 6) -> (100, 6)
  arc A409 (90, 9) -> (90, 6) centre (90, 7.5) ccw
  arc A410 (120, 6) -> (120, 9) centre (120, 7.5) ccw
  line L419 (120, 9) -> (110, 9)
  line L420 (110, 6) -> (120, 6)
  arc A411 (110, 9) -> (110, 6) centre (110, 7.5) ccw
  arc A412 (140, 6) -> (140, 9) centre (140, 7.5) ccw
  line L421 (140, 9) -> (130, 9)
  line L422 (130, 6) -> (140, 6)
  arc A413 (130, 9) -> (130, 6) centre (130, 7.5) ccw
  arc A414 (160, 6) -> (160, 9) centre (160, 7.5) ccw
  line L423 (160, 9) -> (150, 9)
  line L424 (150, 6) -> (160, 6)
  arc A415 (150, 9) -> (150, 6) centre (150, 7.5) ccw
  arc A416 (180, 6) -> (180, 9) centre (180, 7.5) ccw
  line L425 (180, 9) -> (170, 9)
  line L426 (170, 6) -> (180, 6)
  arc A417 (170, 9) -> (170, 6) centre (170, 7.5) ccw
  arc A418 (200, 6) -> (200, 9) centre (200, 7.5) ccw
  line L427 (200, 9) -> (190, 9)
  line L428 (190, 6) -> (200, 6)
  arc A419 (190, 9) -> (190, 6) centre (190, 7.5) ccw
  arc A420 (100, 16) -> (100, 19) centre (100, 17.5) ccw
  line L429 (100, 19) -> (90, 19)
  line L430 (90, 16) -> (100, 16)
  arc A421 (90, 19) -> (90, 16) centre (90, 17.5) ccw
  arc A422 (120, 16) -> (120, 19) centre (120, 17.5) ccw
  line L431 (120, 19) -> (110, 19)
  line L432 (110, 16) -> (120, 16)
  arc A423 (110, 19) -> (110, 16) centre (110, 17.5) ccw
  arc A424 (140, 16) -> (140, 19) centre (140, 17.5) ccw
  line L433 (140, 19) -> (130, 19)
  line L434 (130, 16) -> (140, 16)
  arc A425 (130, 19) -> (130, 16) centre (130, 17.5) ccw
  arc A426 (160, 16) -> (160, 19) centre (160, 17.5) ccw
  line L435 (160, 19) -> (150, 19)
  line L436 (150, 16) -> (160, 16)
  arc A427 (150, 19) -> (150, 16) centre (150, 17.5) ccw
  arc A428 (180, 16) -> (180, 19) centre (180, 17.5) ccw
  line L437 (180, 19) -> (170, 19)
  line L438 (170, 16) -> (180, 16)
  arc A429 (170, 19) -> (170, 16) centre (170, 17.5) ccw
  arc A430 (200, 16) -> (200, 19) centre (200, 17.5) ccw
  line L439 (200, 19) -> (190, 19)
  line L440 (190, 16) -> (200, 16)
  arc A431 (190, 19) -> (190, 16) centre (190, 17.5) ccw
  arc A432 (120, 26) -> (120, 29) centre (120, 27.5) ccw
  line L441 (120, 29) -> (110, 29)
  line L442 (110, 26) -> (120, 26)
  arc A433 (110, 29) -> (110, 26) centre (110, 27.5) ccw
  arc A434 (140, 26) -> (140, 29) centre (140, 27.5) ccw
  line L443 (140, 29) -> (130, 29)
  line L444 (130, 26) -> (140, 26)
  arc A435 (130, 29) -> (130, 26) centre (130, 27.5) ccw
  arc A436 (160, 26) -> (160, 29) centre (160, 27.5) ccw
  line L445 (160, 29) -> (150, 29)
  line L446 (150, 26) -> (160, 26)
  arc A437 (150, 29) -> (150, 26) centre (150, 27.5) ccw
  arc A438 (180, 26) -> (180, 29) centre (180, 27.5) ccw
  line L447 (180, 29) -> (170, 29)
  line L448 (170, 26) -> (180, 26)
  arc A439 (170, 29) -> (170, 26) centre (170, 27.5) ccw
  arc A440 (120, 36) -> (120, 39) centre (120, 37.5) ccw
  line L449 (120, 39) -> (110, 39)
  line L450 (110, 36) -> (120, 36)
  arc A441 (110, 39) -> (110, 36) centre (110, 37.5) ccw
  arc A442 (140, 36) -> (140, 39) centre (140, 37.5) ccw
  line L451 (140, 39) -> (130, 39)
  line L452 (130, 36) -> (140, 36)
  arc A443 (130, 39) -> (130, 36) centre (130, 37.5) ccw
  arc A444 (160, 36) -> (160, 39) centre (160, 37.5) ccw
  line L453 (160, 39) -> (150, 39)
  line L454 (150, 36) -> (160, 36)
  arc A445 (150, 39) -> (150, 36) centre (150, 37.5) ccw
  arc A446 (180, 36) -> (180, 39) centre (180, 37.5) ccw
  line L455 (180, 39) -> (170, 39)
  line L456 (170, 36) -> (180, 36)
  arc A447 (170, 39) -> (170, 36) centre (170, 37.5) ccw
  line L457 (215, -145) -> (190, -190)
  line L458 (190, -190) -> (100, -190)
  line L459 (100, -190) -> (75, -145)
  line L460 (360, -72.5) -> (-31.5578, -72.5) construction
  line L461 (55, 0) -> (75, 0)
  line L462 (100, 45) -> (75, 0)
  line L463 (190, 45) -> (100, 45)
  line L464 (215, 0) -> (190, 45)
  line L465 (29.7917, -27.5) -> (55, 0)
  line L466 (55, -145) -> (75, -145)
  line L467 (215, 0) -> (235, 0)
  line L468 (215, -145) -> (235, -145)
  point P0 (343.5, -56.5)
  point P1 (343.5, -88.5)
  point P2 (20, -56.5)
  point P3 (20, -88.5)
  point P4 (175, -72.5)
  point P5 (115, -182.5)
  point P6 (135, -182.5)
  point P7 (155, -182.5)
  point P8 (175, -182.5)
  point P9 (115, -172.5)
  point P10 (135, -172.5)
  point P11 (155, -172.5)
  point P12 (175, -172.5)
  point P13 (95, -162.5)
  point P14 (115, -162.5)
  point P15 (135, -162.5)
  point P16 (155, -162.5)
  point P17 (175, -162.5)
  point P18 (195, -162.5)
  point P19 (95, -152.5)
  point P20 (115, -152.5)
  point P21 (135, -152.5)
  point P22 (155, -152.5)
  point P23 (175, -152.5)
  point P24 (195, -152.5)
  point P25 (215, -152.5)
  point P26 (95, -142.5)
  point P27 (115, -142.5)
  point P28 (135, -142.5)
  point P29 (155, -142.5)
  point P30 (175, -142.5)
  point P31 (195, -142.5)
  point P32 (55, -132.5)
  point P33 (75, -132.5)
  point P34 (95, -132.5)
  point P35 (115, -132.5)
  point P36 (135, -132.5)
  point P37 (155, -132.5)
  point P38 (175, -132.5)
  point P39 (195, -132.5)
  point P40 (215, -132.5)
  point P41 (235, -132.5)
  point P42 (35, -122.5)
  point P43 (55, -122.5)
  point P44 (75, -122.5)
  point P45 (95, -122.5)
  point P46 (115, -122.5)
  point P47 (135, -122.5)
  point P48 (155, -122.5)
  point P49 (175, -122.5)
  point P50 (195, -122.5)
  point P51 (215, -122.5)
  point P52 (235, -122.5)
  point P53 (255, -122.5)
  point P54 (55, -112.5)
  point P55 (75, -112.5)
  point P56 (95, -112.5)
  point P57 (115, -112.5)
  point P58 (135, -112.5)
  point P59 (155, -112.5)
  point P60 (175, -112.5)
  point P61 (195, -112.5)
  point P62 (215, -112.5)
  point P63 (235, -112.5)
  point P64 (255, -112.5)
  point P65 (275, -112.5)
  point P66 (15, -102.5)
  point P67 (55, -102.5)
  point P68 (75, -102.5)
  point P69 (95, -102.5)
  point P70 (115, -102.5)
  point P71 (135, -102.5)
  point P72 (155, -102.5)
  point P73 (175, -102.5)
  point P74 (195, -102.5)
  point P75 (215, -102.5)
  point P76 (235, -102.5)
  point P77 (255, -102.5)
  point P78 (275, -102.5)
  point P79 (295, -102.5)
  point P80 (315, -102.5)
  point P81 (55, -92.5)
  point P82 (75, -92.5)
  point P83 (95, -92.5)
  point P84 (115, -92.5)
  point P85 (135, -92.5)
  point P86 (155, -92.5)
  point P87 (175, -92.5)
  point P88 (195, -92.5)
  point P89 (215, -92.5)
  point P90 (235, -92.5)
  point P91 (255, -92.5)
  point P92 (275, -92.5)
  point P93 (295, -92.5)
  point P94 (315, -92.5)
  point P95 (55, -82.5)
  point P96 (75, -82.5)
  point P97 (95, -82.5)
  point P98 (115, -82.5)
  point P99 (135, -82.5)
  point P100 (155, -82.5)
  point P101 (175, -82.5)
  point P102 (195, -82.5)
  point P103 (215, -82.5)
  point P104 (235, -82.5)
  point P105 (255, -82.5)
  point P106 (275, -82.5)
  point P107 (295, -82.5)
  point P108 (315, -82.5)
  point P109 (35, -72.5)
  point P110 (55, -72.5)
  point P111 (75, -72.5)
  point P112 (95, -72.5)
  point P113 (115, -72.5)
  point P114 (135, -72.5)
  point P115 (155, -72.5)
  point P116 (195, -72.5)
  point P117 (215, -72.5)
  point P118 (235, -72.5)
  point P119 (255, -72.5)
  point P120 (275, -72.5)
  point P121 (295, -72.5)
  point P122 (315, -72.5)
  point P123 (55, -62.5)
  point P124 (75, -62.5)
  point P125 (95, -62.5)
  point P126 (115, -62.5)
  point P127 (135, -62.5)
  point P128 (155, -62.5)
  point P129 (175, -62.5)
  point P130 (195, -62.5)
  point P131 (215, -62.5)
  point P132 (235, -62.5)
  point P133 (255, -62.5)
  point P134 (275, -62.5)
  point P135 (295, -62.5)
  point P136 (315, -62.5)
  point P137 (55, -52.5)
  point P138 (75, -52.5)
  point P139 (95, -52.5)
  point P140 (115, -52.5)
  point P141 (135, -52.5)
  point P142 (155, -52.5)
  point P143 (175, -52.5)
  point P144 (195, -52.5)
  point P145 (215, -52.5)
  point P146 (235, -52.5)
  point P147 (255, -52.5)
  point P148 (275, -52.5)
  point P149 (295, -52.5)
  point P150 (315, -52.5)
  point P151 (15, -42.5)
  point P152 (35, -42.5)
  point P153 (55, -42.5)
  point P154 (75, -42.5)
  point P155 (95, -42.5)
  point P156 (115, -42.5)
  point P157 (135, -42.5)
  point P158 (155, -42.5)
  point P159 (175, -42.5)
  point P160 (195, -42.5)
  point P161 (215, -42.5)
  point P162 (235, -42.5)
  point P163 (255, -42.5)
  point P164 (275, -42.5)
  point P165 (295, -42.5)
  point P166 (315, -42.5)
  point P167 (55, -32.5)
  point P168 (75, -32.5)
  point P169 (95, -32.5)
  point P170 (115, -32.5)
  point P171 (135, -32.5)
  point P172 (155, -32.5)
  point P173 (175, -32.5)
  point P174 (195, -32.5)
  point P175 (215, -32.5)
  point P176 (235, -32.5)
  point P177 (255, -32.5)
  point P178 (275, -32.5)
  point P179 (55, -22.5)
  point P180 (75, -22.5)
  point P181 (95, -22.5)
  point P182 (115, -22.5)
  point P183 (135, -22.5)
  point P184 (155, -22.5)
  point P185 (175, -22.5)
  point P186 (195, -22.5)
  point P187 (215, -22.5)
  point P188 (235, -22.5)
  point P189 (255, -22.5)
  point P190 (55, -12.5)
  point P191 (75, -12.5)
  point P192 (95, -12.5)
  point P193 (115, -12.5)
  point P194 (135, -12.5)
  point P195 (155, -12.5)
  point P196 (175, -12.5)
  point P197 (195, -12.5)
  point P198 (215, -12.5)
  point P199 (235, -12.5)
  point P200 (95, -2.5)
  point P201 (115, -2.5)
  point P202 (135, -2.5)
  point P203 (155, -2.5)
  point P204 (175, -2.5)
  point P205 (195, -2.5)
  point P206 (95, 7.5)
  point P207 (115, 7.5)
  point P208 (135, 7.5)
  point P209 (155, 7.5)
  point P210 (175, 7.5)
  point P211 (195, 7.5)